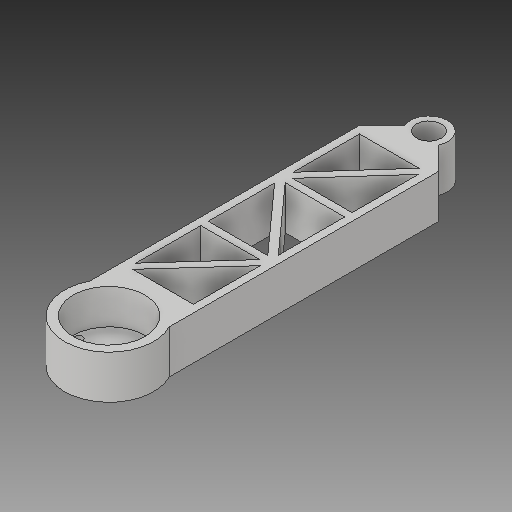
# Autodesk Inventor part: leg 3.0
Saved by Autodesk Inventor 2018.2 (Build 222227000, 227)
## iProperties
Created: 2018-03-10
Part Number: leg 3.0
Material: Generic
Document SubType Name: Modeling
Designer: MIABo
Density: 1 g/cm^3
Appearance: Default
Author: MIABo
## iProperties of the stored document leg 2_3DPrint.ipt
Created: 2018-03-10
Part Number: leg 2_3DPrint
Material: Generic
Document SubType Name: Modeling
Designer: MIABo
Density: 1 g/cm^3
Appearance: Default
Author: MIABo
Autodesk Inventor part; units mm, degrees
ref_plane "YZ Plane" through (0, 0, 0) normal (1, 0, 0) x (0, 1, 0)
ref_plane "XZ Plane" through (0, 0, 0) normal (0, 1, 0) x (-1, 0, 0)
ref_plane "XY Plane" through (0, 0, 0) normal (0, 0, 1) x (1, 0, 0)
sketch "Sketch1" plane through (0, 0, 0) normal (0, 1, 0) x (-1, 0, 0)
  circle A0 centre (0, 0) radius 22.86
  line L0 (14.5416, -26.67) -> (-16.51, -26.67)
  line L1 (-20.32, -15.24) -> (-20.32, -55.88)
  line L2 (-13.6865, -63.5) -> (16.51, -63.5)
  line L3 (20.32, -55.88) -> (20.32, -15.24)
  line L4 (16.51, -67.31) -> (-16.51, -67.31)
  line L5 (-20.32, -59.69) -> (-20.32, -100.33)
  line L6 (-16.51, -104.14) -> (13.9515, -104.14)
  line L7 (20.32, -100.33) -> (20.32, -59.69)
  line L8 (13.9515, -107.95) -> (-16.51, -107.95)
  line L9 (-20.32, -104.14) -> (-20.32, -144.78)
  line L10 (20.32, -144.78) -> (20.32, -104.14)
  line L11 (20.32, -15.24) -> (20.32, -10.4727)
  circle A1 centre (0, -163.83) radius 6.35
  line L12 (-20.32, -15.24) -> (-20.32, -10.4727)
  line L13 (20.32, -55.88) -> (20.32, -59.69)
  line L14 (20.32, -100.33) -> (20.32, -104.14)
  line L15 (-20.32, -55.88) -> (-20.32, -59.69)
  line L16 (-20.32, -100.33) -> (-20.32, -104.14)
  line L17 (20.32, -144.78) -> (20.32, -148.59)
  line L18 (-20.32, -144.78) -> (-20.32, -148.59)
  line L19 (20.32, -148.59) -> (8.7779, -160.1321)
  line L20 (-20.32, -148.59) -> (-8.7779, -160.1321)
  line L21 (16.51, -30.1719) -> (16.51, -63.5)
  line L22 (-16.51, -26.67) -> (-16.51, -60.9418)
  line L23 (16.51, -67.31) -> (16.51, -101.2863)
  line L24 (-16.51, -67.31) -> (-16.51, -104.14)
  line L25 (16.51, -110.8037) -> (16.51, -144.78)
  line L26 (-16.51, -141.9263) -> (-16.51, -107.95)
  arc A2 (-8.7779, -160.1321) -> (8.7779, -160.1321) centre (0, -163.83) ccw
  line L27 (14.5416, -26.67) -> (-16.51, -60.9418)
  line L28 (16.9388, -26.8614) -> (16.51, -27.3347)
  line L29 (17.3651, -29.2282) -> (-13.6865, -63.5)
  line L30 (-13.9515, -67.31) -> (16.51, -101.2863)
  line L31 (-16.51, -70.1637) -> (13.9515, -104.14)
  line L32 (13.9515, -107.95) -> (-16.51, -141.9263)
  line L33 (16.51, -110.8037) -> (-13.9515, -144.78)
  line L34 (-19.0685, -144.78) -> (-16.51, -144.78)
  line L35 (-13.9515, -144.78) -> (16.51, -144.78)
  dimension "d0" = 45.72
  dimension "d2" = 26.67
  dimension "d3" = 36.83
  dimension "d5" = 20.32
  dimension "d6" = 3.81
  dimension "d7" = 40.64
  dimension "d8" = 3.81
  dimension "d10" = 12.7
  dimension "d11" = 3.81
  dimension "d12" = 3.81
  dimension "d13" = 135
  dimension "d14" = 3.81
  dimension "d15" = 3.81
  dimension "d16" = 3.81
  dimension "d17" = 36.83
  dimension "d19" = 94.2927
  dimension "d20" = 62.8618
  dimension "d21" = 123.0295
  dimension "d22" = 94.2927
  dimension "d23" = 91.5986
  dimension "d24" = 62.8618
  dimension "d25" = 3.81
  dimension "d26" = 36.83
  dimension "d27" = 65.5559
  dimension "d28" = 60.1677
  dimension "d29" = 19.05
  dimension "d32" = 1.905
  dimension "d37" = 42.178
  dimension "d38" = 138.122
  dimension "d39" = 138.122
  dimension "d40" = 118.11
  dimension "d41" = 36.83
  dimension "d42" = 0
  dimension "d43" = 3.81
  dimension "d44" = 3.81
  dimension "d45" = 86.2593
  dimension "d46" = 55.3203
  dimension "d47" = 3.3812
  dimension "d48" = 11.5421
  dimension "d49" = 36.83
  dimension "d50" = 119.4374
  dimension "d51" = 119.4374
  dimension "d52" = 20.32
  constraints: 72 end point, 12 parallel, 8 collinear, 8 perpendicular, 7 point on line, 4 point on circle, 4 vertical, 3 centre point, 3 horizontal, 2 coincident, 2 symmetric about line
  measures "d0" diameter of A0
  measures "d2" distance from line of L0 point (0, 0)
  measures "d3" distance between parallel lines of L2 L0
  measures "d5" distance from line of point (0, 0) L3
  measures "d6" distance between parallel lines of L4 L2
  measures "d7" distance between parallel lines of L1 L3
  measures "d8" distance between parallel lines of L8 L6
  measures "d10" diameter of A1
  measures "d11" distance of L9.end L18.end
  measures "d12" distance of L10.start L17.end
  measures "d13" angle of L19 L17
  measures "d14" distance between parallel lines of L3 L21
  measures "d15" distance between parallel lines of L1 L22
  measures "d16" distance between parallel lines of L23 L11
  measures "d17" distance between parallel lines of L24 L11
  measures "d19" distance from line of L3.end L19
  measures "d20" distance from line of L7.end L19
  measures "d21" distance from line of L1.start L19
  measures "d22" distance from line of L1.end L19
  measures "d23" distance from line of L5.start L19
  measures "d24" distance from line of L5.end L19
  measures "d25" distance between parallel lines of L11 L25
  measures "d26" distance between parallel lines of L26 L11
  measures "d27" distance from line of L3.start L19
  measures "d28" distance from line of L9.start L19
  measures "d29" diameter of A2
  measures "d32" distance between parallel lines of L28 L27
  measures "d37" angle of L29 L13
  measures "d38" angle of L33 L13
  measures "d39" angle of L17 L30
  measures "d40" distance between parallel lines of L35 L0
  measures "d41" distance between parallel lines of L8 L35
  measures "d42" distance between parallel lines of L34 L35
  measures "d43" distance between parallel lines of L32 L33
  measures "d44" distance between parallel lines of L31 L30
  measures "d45" distance from line of point (0, 0) L33
  measures "d46" distance from line of point (0, 0) L30
  measures "d47" distance from line of L28.start L11
  measures "d48" distance from line of L19.end L11
  measures "d49" distance from line of L34.end L11
  measures "d50" distance from line of point (0, 0) L19
  measures "d51" distance from line of point (0, 0) L20
  measures "d52" distance from line of A2.centre L11
extrude "Extrusion1" add sketch "Sketch1" along normal blind 22.225
sketch "Sketch2" plane through (0, 22.225, 0) normal (0, 1, 0) x (1, 0, 0)
  circle A0 centre (0, 0) radius 18.415
  dimension "d55" = 36.83
  constraints: 1 centre point, 1 coincident
  measures "d55" diameter of A0
extrude "Extrusion2" cut sketch "Sketch2" against normal blind 17.907
sketch "Sketch3" plane through (0, 4.318, 0) normal (0, 1, 0) x (1, 0, 0)
  circle A0 centre (0, -6.985) radius 6.096
  line L0 (0, 0) -> (0, -18.9723)
  arc A1 (-20.32, 10.4727) -> (20.32, 10.4727) centre (0, 0) ccw projected
  line L1 (-15.494, 0) -> (15.494, 0)
  circle A2 centre (-15.494, 0) radius 1.9939
  circle A3 centre (15.494, 0) radius 1.9939
  point P0 (0, -22.86)
  dimension "d58" = 6.985
  dimension "d59" = 12.192
  dimension "d61" = 3.9878
  dimension "d62" = 30.988
  dimension "d63" = 15.494
  dimension "d65" = 18.9722
  constraints: 5 end point, 3 centre point, 2 point on line, 1 coincident, 1 equal radius, 1 horizontal, 1 midpoint, 1 point on circle, 1 vertical
  measures "d58" distance of L0.start A0.centre
  measures "d59" diameter of A0
  measures "d61" diameter of A2
  measures "d62" distance of L1.end L1.start
  measures "d63" distance of L1.start L0.start
  measures "d65" distance from line of L0.end L1
extrude "Extrusion3" cut sketch "Sketch3" against normal blind 36.322
body "Solid1"
